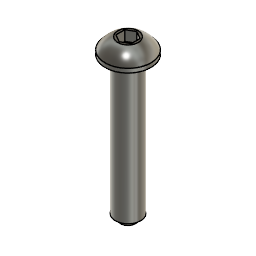
case-accel-lsm6dsv16x-rp2354a (Autodesk Fusion 360 archive; units mm, degrees)
design "HW_M2p5x14-BHCS"
Autodesk Fusion 360 part; units mm, degrees
note: some values were not read from the file. Chosen so that the rebuilt part matches the saved one: a side.
sketch "Sketch1" plane through (0, 0, 0) normal (0, 1, 0) x (1, 0, 0)
  line L0 (0, -1.5) -> (0, 14)
  line L1 (0, 14) -> (0.75, 14)
  line L2 (0.75, 14) -> (1.25, 13.5)
  line L3 (1.25, 13.5) -> (1.25, 0)
  line L4 (1.25, 0) -> (2.25, 0)
  line L5 (2.25, 0) -> (2.25, -0.4)
  line L6 (0, -1.5) -> (1, -1.5)
  arc A0 (1, -1.5) -> (2.25, -0.4) centre (0, 0.8966) ccw
  dimension "d1" = 14
  dimension "d2" = 1.5
  dimension "d3" = 1
  dimension "d4" = 0.4
  dimension "d5" = 2.25
  dimension "d6" = 1.25
  dimension "d7" = 45
  dimension "d8" = 0.5
  constraint vertical L0
  constraint perpendicular L0 L1
  constraint perpendicular L1 L3
  constraint perpendicular L3 L4
  constraint perpendicular L4 L5
  constraint perpendicular L0 L6
  constraint coincident origin L4
  constraint coincident L0 A0.centre
  constraint coincident origin L0
  measures "d1" distance of origin L0.end
  measures "d2" distance of origin L0.start
  measures "d3" distance of L0.start L6.end
  measures "d4" distance of L4.end L5.end
  measures "d5" distance of L0 L4.end
  measures "d6" distance of origin L3
  measures "d7" angle of L1 L2
  measures "d8" distance of L1 L2.end
revolve "Revolve1" add sketch "Sketch1" angle 360 about axis through (0, 0, 1.5) along (0, 0, -1)
sketch "Sketch2" plane through (0, 0, 1.5) normal (0, 0, 1) x (-1, 0, 0)
  circle A0 centre (0, 0) radius 1
  line L0 (-0.75, -0.433) -> (0, -0.866)
  line L1 (0, -0.866) -> (0.75, -0.433)
  line L2 (0.75, -0.433) -> (0.75, 0.433)
  line L3 (0.75, 0.433) -> (0, 0.866)
  line L4 (0, 0.866) -> (-0.75, 0.433)
  line L5 (-0.75, 0.433) -> (-0.75, -0.433)
  dimension "d10" = 1.5
  constraint coincident A0.centre origin
  constraint vertical L2
  measures "d10" distance of L1.end L5
extrude "Extrude1" cut sketch "Sketch2" against normal up to surface (1 mm away) contours L0 L1 L2 L3 L4 L5
equation "d5 = ( 4.5 / 2 ) * 1 mm"
equation "d6 = ( 2.5 / 2 ) * 1 mm"

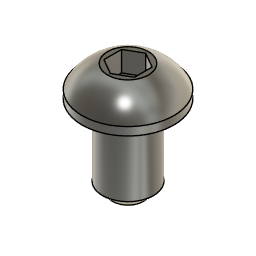
design "HW_M2p5x4-BHCS"
Autodesk Fusion 360 part; units mm, degrees
sketch "Sketch1" plane through (0, 0, 0) normal (0, 1, 0) x (1, 0, 0)
  line L0 (0, -1.5) -> (0, 4)
  line L1 (0, 4) -> (0.75, 4)
  line L2 (0.75, 4) -> (1.25, 3.5)
  line L3 (1.25, 3.5) -> (1.25, 0)
  line L4 (1.25, 0) -> (2.25, 0)
  line L5 (2.25, 0) -> (2.25, -0.4)
  line L6 (0, -1.5) -> (1, -1.5)
  arc A0 (1, -1.5) -> (2.25, -0.4) centre (0, 0.8966) ccw
  dimension "d1" = 4
  dimension "d2" = 1.5
  dimension "d3" = 1
  dimension "d4" = 0.4
  dimension "d5" = 2.25
  dimension "d6" = 1.25
  dimension "d7" = 45
  dimension "d8" = 0.5
  constraint vertical L0
  constraint perpendicular L0 L1
  constraint perpendicular L1 L3
  constraint perpendicular L3 L4
  constraint perpendicular L4 L5
  constraint perpendicular L0 L6
  constraint coincident origin L4
  constraint coincident L0 A0.centre
  constraint coincident origin L0
  measures "d1" distance of origin L0.end
  measures "d2" distance of origin L0.start
  measures "d3" distance of L0.start L6.end
  measures "d4" distance of L4.end L5.end
  measures "d5" distance of L0 L4.end
  measures "d6" distance of origin L3
  measures "d7" angle of L1 L2
  measures "d8" distance of L1 L2.end
revolve "Revolve1" add sketch "Sketch1" angle 360 about axis through (0, 0, 1.5) along (0, 0, -1)
sketch "Sketch2" plane through (0, 0, 1.5) normal (0, 0, 1) x (-1, 0, 0)
  circle A0 centre (0, 0) radius 1
  line L0 (-0.75, -0.433) -> (0, -0.866)
  line L1 (0, -0.866) -> (0.75, -0.433)
  line L2 (0.75, -0.433) -> (0.75, 0.433)
  line L3 (0.75, 0.433) -> (0, 0.866)
  line L4 (0, 0.866) -> (-0.75, 0.433)
  line L5 (-0.75, 0.433) -> (-0.75, -0.433)
  dimension "d10" = 1.5
  constraint coincident A0.centre origin
  constraint vertical L2
  measures "d10" distance of L1.end L5
extrude "Extrude1" cut sketch "Sketch2" against normal up to surface (1 mm away) contours L0 L1 L2 L3 L4 L5
equation "d5 = ( 4.5 / 2 ) * 1 mm"
equation "d6 = ( 2.5 / 2 ) * 1 mm"

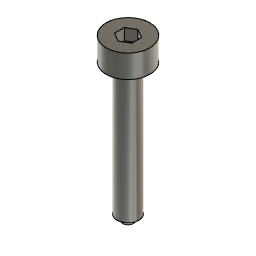
design "HW_M2x12-SHCS"
Autodesk Fusion 360 part; units mm, degrees
sketch "Sketch1" plane through (0, 0, 0) normal (0, 1, 0) x (1, 0, 0)
  line L0 (0, -2) -> (0, 12)
  line L1 (0, 12) -> (0.45, 12)
  line L2 (0.45, 12) -> (0.95, 11.5)
  line L3 (0.95, 11.5) -> (0.95, 0)
  line L4 (0.95, 0) -> (1.9, 0)
  line L5 (1.9, 0) -> (1.9, -2)
  line L6 (1.9, -2) -> (0, -2)
  dimension "d1" = 12
  dimension "d2" = 45
  dimension "d3" = 0.5
  dimension "d4" = 0.95
  dimension "d5" = 2
  dimension "d6" = 1.9
  constraint vertical L0
  constraint perpendicular L0 L1
  constraint perpendicular L1 L3
  constraint perpendicular L3 L4
  constraint perpendicular L4 L5
  constraint horizontal L6
  constraint coincident origin L0
  constraint coincident origin L4
  measures "d1" distance of origin L1
  measures "d2" angle of L1 L2
  measures "d3" horizontal distance of L1.end L2.end
  measures "d4" distance of L0.end L3
  measures "d5" distance of L4.end L5.end
  measures "d6" distance of L0.start L5.end
revolve "Revolve1" add sketch "Sketch1" angle 360 about axis through (0, 0, 2) along (0, 0, -1)
sketch "Sketch2" plane through (0, 0, 2) normal (0, 0, 1) x (-1, 0, 0)
  circle A0 centre (0, 0) radius 1.9
  line L0 (-0.75, -0.433) -> (0, -0.866)
  line L1 (0, -0.866) -> (0.75, -0.433)
  line L2 (0.75, -0.433) -> (0.75, 0.433)
  line L3 (0.75, 0.433) -> (0, 0.866)
  line L4 (0, 0.866) -> (-0.75, 0.433)
  line L5 (-0.75, 0.433) -> (-0.75, -0.433)
  dimension "d8" = 1.5
  constraint coincident A0.centre origin
  constraint vertical L5
  measures "d8" distance of L1.end L5
extrude "Extrude1" cut sketch "Sketch2" against normal blind 1 contours L0 L1 L2 L3 L4 L5
equation "d4 = ( 1.9 / 2 ) * 1 mm"
equation "d6 = ( 3.8 / 2 ) * 1 mm"
